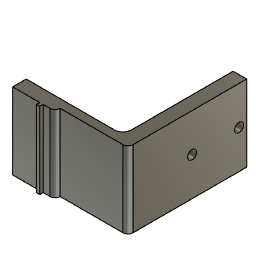
droy-topangle v5 (Autodesk Fusion 360 design; units mm, degrees)
Autodesk Fusion 360 part; units mm, degrees
note: some values were not read from the file. Set by a fixed rule: which sketch regions a step uses.
sketch "Sketch1" plane through (0, 0, 0) normal (0, 0, 1) x (1, 0, 0)
  line L0 (0, 0) -> (65, 0)
  line L1 (65, 0) -> (65, 8)
  line L2 (65, 8) -> (0, 8)
  line L3 (0, 8) -> (0, 0)
  line L4 (65, 0) -> (57, 0)
  line L5 (57, 0) -> (57, 73)
  line L6 (57, 73) -> (65, 73)
  line L7 (65, 73) -> (65, 0)
  line L8 (65, 0) -> (25, 0)
  line L9 (25, 0) -> (25, 3)
  line L10 (25, 3) -> (65, 3)
  line L11 (65, 3) -> (65, 0)
  dimension "d1" = 65
  dimension "d2" = 8
  dimension "d3" = 8
  dimension "d4" = 73
  dimension "d37" = 40
  dimension "d38" = 3
  constraint horizontal L0
  constraint vertical L1
  constraint horizontal L2
  constraint vertical L3
  constraint coincident L0.start L3.end
  constraint horizontal L4
  constraint vertical L5
  constraint horizontal L6
  constraint vertical L7
  constraint horizontal L8
  constraint vertical L9
  constraint horizontal L10
  constraint vertical L11
  measures "d1" distance of L0.start L0.end
  measures "d2" distance of L0.start L2.end
  measures "d3" distance of L0.end L4.end
  measures "d4" distance of L0.end L6.end
  measures "d37" distance of L0.end L8.end
  measures "d38" distance of L0.end L10.end
extrude "Extrude1" add sketch "Sketch1" along normal blind 45
sketch "Sketch2" plane through (0, 0, 0) normal (0, -1, 0) x (1, 0, 0)
  line L0 (0, 0) -> (65, 0)
  line L1 (65, 0) -> (65, 45)
  line L2 (65, 45) -> (0, 45)
  line L3 (0, 45) -> (0, 0)
  line L4 (16, 0) -> (18, 0)
  line L5 (18, 0) -> (18, 60)
  line L6 (18, 60) -> (16, 60)
  line L7 (16, 60) -> (16, 0)
  dimension "d7" = 2
  dimension "d8" = 60
  dimension "d9" = 16
  constraint horizontal L4
  constraint vertical L5
  constraint horizontal L6
  constraint vertical L7
  constraint coincident L0 L4.start
  measures "d7" distance of L4.start L4.end
  measures "d8" distance of L4.start L6.end
  measures "d9" distance of L3 L7
extrude "Extrude2" add sketch "Sketch2" along normal blind 2 contours L0 L2 L4 L5 L7
sketch "Sketch3" plane through (57, 0, 0) normal (-1, 0, 0) x (0, -1, 0)
  line L0 (-73, 0) -> (-8, 0)
  line L1 (-8, 0) -> (-8, 45)
  line L2 (-8, 45) -> (-73, 45)
  line L3 (-73, 45) -> (-73, 0)
  line L4 (-73, 22.5) -> (-8.58, 22.5) construction
  circle A0 centre (-68.5, 22.5) radius 2
  circle A1 centre (-40.79, 22.5) radius 2
  circle A2 centre (-68.5, 22.5) radius 2.65
  circle A3 centre (-40.79, 22.5) radius 2.65
  line L5 (-73, 0) -> (-18, 0)
  line L6 (-18, 0) -> (-18, 10)
  line L7 (-18, 10) -> (-73, 10)
  line L8 (-73, 10) -> (-73, 0)
  dimension "d25" = 4
  dimension "d27" = 4
  dimension "d28" = 4.5
  dimension "d29" = 27.71
  dimension "d30" = 5.3
  dimension "d31" = 5.3
  dimension "d49" = 55
  dimension "d50" = 10
  constraint midpoint L3 L4.start
  constraint perpendicular L1 L4
  constraint coincident L4 A0.centre
  constraint midpoint L4 A1.centre
  constraint concentric A0 A2
  constraint concentric A1 A3
  constraint horizontal L5
  constraint vertical L6
  constraint horizontal L7
  constraint vertical L8
  constraint coincident L0.start L3.end
  measures "d25" diameter of A0
  measures "d27" diameter of A1
  measures "d28" distance of L3 A0.centre
  measures "d29" distance of A0.centre A1.centre
  measures "d30" diameter of A2
  measures "d31" diameter of A3
  measures "d49" distance of L0.start L5.end
  measures "d50" distance of L0.start L7.end
extrude "Extrude5" cut sketch "Sketch3" against normal blind 8 contours A0 | A1
extrude "Extrude6" cut sketch "Sketch3" against normal blind 8 contours A2 | A3
extrude "Extrude7" cut sketch "Sketch1" along normal blind 70 contours L0 L5 L8 L9 L10 | L0 L1 L4 L5 L7 L8 L10 L11
fillet "Fillet1" radius 3 1 edges at (25, 0, 22.5)
fillet "Fillet2" radius 3 1 edges at (65, 3, 22.5)
fillet "Fillet3" radius 5 1 edges at (57, 8, 22.5)
equation "d1 = 39 mm + 5 mm + 16 mm + 5 mm"
equation "d4 = 48 mm + 5 mm + 10 mm + 10 mm"
